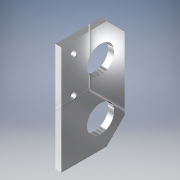
# Autodesk Inventor part: 15102898-16-P-0302
Saved by Autodesk Inventor 2017 (Build 210142000, 142)
## iProperties
Created: 2016-10-02
Part Number: 15102898-16-P-0302
Material: Aluminum 6061
Document SubType Name: Modeling
Designer: gus
Density: 2.7 g/cm^3
Appearance: Aluminum - Flat
Author: gus
Autodesk Inventor part; units mm, degrees
ref_plane "YZ Plane" through (0, 0, 0) normal (1, 0, 0) x (0, 1, 0)
ref_plane "XZ Plane" through (0, 0, 0) normal (0, 1, 0) x (-1, 0, 0)
ref_plane "XY Plane" through (0, 0, 0) normal (0, 0, 1) x (1, 0, 0)
sketch "Sketch1" plane through (0, 0, 0) normal (1, 0, 0) x (0, 1, 0)
  line L0 (0, 0) -> (63.5, 0)
  line L1 (63.5, 0) -> (63.5, -47.625)
  line L2 (63.5, -47.625) -> (44.45, -66.675)
  line L3 (44.45, -66.675) -> (19.05, -66.675)
  circle A0 centre (31.75, -41.275) radius 14.2875
  line L4 (63.5, -25.4) -> (0, -25.4) construction
  circle A1 centre (50.8, -12.7) radius 3.175
  circle A2 centre (12.7, -12.7) radius 3.175
  line L5 (19.05, -66.675) -> (-31.75, -66.675)
  line L6 (-31.75, -66.675) -> (-50.8, -47.625)
  line L7 (-50.8, -47.625) -> (-50.8, 0)
  line L8 (-50.8, 0) -> (0, 0)
  circle A3 centre (-22.225, -41.275) radius 14.2875
  dimension "d0" = 47.625
  dimension "d1" = 28.575
  dimension "d2" = 63.5
  dimension "d4" = 25.4
  dimension "d5" = 31.75
  dimension "d6" = 25.4
  dimension "d7" = 6.35
  dimension "d8" = 6.35
  dimension "d9" = 12.7
  dimension "d10" = 12.7
  dimension "d12" = 12.7
  dimension "d15" = 50.8
  dimension "d16" = 19.05
  dimension "d17" = 25.4
  dimension "d18" = 50.8
  dimension "d19" = 63.5
  dimension "d20" = 41.275
  dimension "d21" = 28.575
  constraints: 18 end point, 4 centre point, 3 perpendicular, 2 equal length, 2 horizontal, 1 equal radius, 1 parallel, 1 point on line
  measures "d0" distance of L0.end L1.end
  measures "d1" diameter of A0
  measures "d2" distance of L0.start L0.end
  measures "d4" distance from line of L3 A0.centre
  measures "d5" distance from line of L1 A0.centre
  measures "d6" distance between parallel lines of L0 L4
  measures "d7" diameter of A1
  measures "d8" diameter of A2
  measures "d9" distance from line of L4 A2.centre
  measures "d10" distance from line of L4 A1.centre
  measures "d12" distance from line of L1 A1.centre
  measures "d15" distance of L3.end L5.end
  measures "d16" distance from line of L5 L6.end
  measures "d17" distance of L2.end L3.end
  measures "d18" distance from line of L0.start L7
  measures "d19" distance from line of L7 A2.centre
  measures "d20" distance from line of L8 A3.centre
  measures "d21" distance from line of L7 A3.centre
extrude "Extrusion1" add sketch "Sketch1" along normal blind 6.35 contours L0 L1 L2 L3 L5 L6 L7 L8 | A3
extrude "Extrusion2" cut sketch "Sketch1" along normal blind 25.4 contours A3
body "Solid1"
